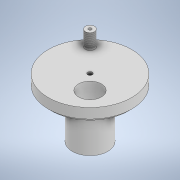
# Autodesk Inventor part: TopReactor
Saved by Autodesk Inventor 2022 (Build 260153070, 153G)
## iProperties
Created: 2021-07-20
Part Number: TopReactor
Material: Generic
Document SubType Name: Modeling
Designer: Eakawit_kor
Density: 1 g/cm^3
Appearance: Default
Author: Eakawit_kor
Autodesk Inventor part; units mm, degrees
ref_plane "YZ Plane" through (0, 0, 0) normal (1, 0, 0) x (0, 1, 0)
ref_plane "XZ Plane" through (0, 0, 0) normal (0, 1, 0) x (-1, 0, 0)
ref_plane "XY Plane" through (0, 0, 0) normal (0, 0, 1) x (1, 0, 0)
sketch "Sketch1" plane through (0, 0, 0) normal (0, 1, 0) x (-1, 0, 0)
  circle A0 centre (0, 0) radius 25
  dimension "d0" = 50
  constraints: 1 centre point, 1 coincident
  measures "d0" diameter of A0
extrude "Extrusion1" add sketch "Sketch1" along normal blind 2
sketch "Sketch3" plane through (0, 2, 0) normal (0, 1, 0) x (1, 0, 0)
  circle A0 centre (0, 0) radius 27
  circle A1 centre (0, 0) radius 25 projected
  dimension "d3" = 2
  constraints: 1 centre point, 1 coincident
  measures "d3" radial gap between concentric circles of A0 A1
extrude "Extrusion2" add sketch "Sketch3" along normal blind 6.5 contours A0 | A1
sketch "Sketch4" plane through (0, 8.5, 0) normal (0, 1, 0) x (1, 0, 0)
  circle A0 centre (0, 0) radius 1.5
  circle A1 centre (-15, 15) radius 1
  dimension "d6" = 3
  dimension "d8" = 15
  dimension "d9" = 15
  dimension "d10" = 2
  constraints: 2 centre point, 1 coincident
  measures "d6" diameter of A0
  measures "d8" horizontal distance of point (0, 0) A1.centre
  measures "d9" horizontal distance of point (0, 0) A1.centre
  measures "d10" diameter of A1
extrude "Extrusion3" cut sketch "Sketch4" against normal through all
sketch "Sketch5" plane through (0, 8.5, 0) normal (0, 1, 0) x (1, 0, 0)
  circle A0 centre (-15, 15) radius 3
  circle A1 centre (-15, 15) radius 1 projected
  point P0 (0, 0)
  dimension "d14" = 2
  constraints: 1 centre point, 1 concentric
  measures "d14" radial gap between concentric circles of A1 A0
extrude "Extrusion4" add sketch "Sketch5" along normal blind 10
thread "Thread1" size "M6x1" class "6g" standard "ANSI Metric M Profile" length 9
sketch "Sketch10" plane through (0, 0, 0) normal (0, -1, 0) x (1, 0, 0)
  circle A0 centre (9.5, 9.5) radius 11.5
  point P0 (0, 0)
  dimension "d31" = 23
  dimension "d32" = 9.5
  dimension "d33" = 9.5
  constraints: 1 centre point
  measures "d31" diameter of A0
  measures "d32" horizontal distance of point (0, 0) A0.centre
  measures "d33" horizontal distance of point (0, 0) A0.centre
extrude "Extrusion8" add sketch "Sketch10" along normal blind 20
sketch "Sketch11" plane through (9.5, -20, 9.5) normal (0, -1, 0) x (1, 0, 0)
  circle A0 centre (0, 0) radius 10.6
  circle A1 centre (0, 0) radius 11.5 projected
  point P0 (-9.5, -9.5)
  dimension "d36" = 21.2
  constraints: 1 centre point, 1 concentric
  measures "d36" diameter of A0
extrude "Extrusion9" cut sketch "Sketch11" against normal blind 2.5 contours A0
sketch "Sketch12" plane through (9.5, -17.5, 9.5) normal (0, -1, 0) x (1, 0, 0)
  circle A0 centre (0, 0) radius 7.4
  circle A1 centre (0, 0) radius 10.6 projected
  point P0 (-9.5, -9.5)
  dimension "d39" = 14.8
  constraints: 1 centre point, 1 concentric
  measures "d39" diameter of A0
extrude "Extrusion10" cut sketch "Sketch12" against normal through all contours A0
thread "Thread2" size "M15x1.5" class "6H" standard "ANSI Metric M Profile" length 9
body "Solid1"
